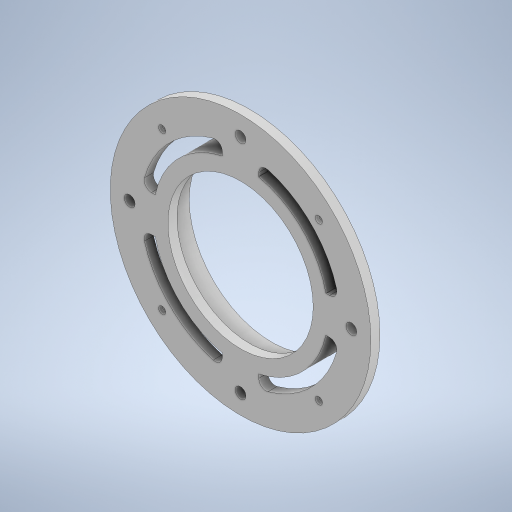
# Autodesk Inventor part: 하단 맨 위부분
Saved by Autodesk Inventor 2023 (Build 270158000, 158)
## iProperties
Created: 2022-06-06
Part Number: 하단 맨 위부분
Material: 일반
Document SubType Name: Modeling
Designer: fly01
Density: 1 g/cm^3
Appearance: 기본값
Author: fly01
Autodesk Inventor part; units mm, degrees
ref_plane "YZ Plane" through (0, 0, 0) normal (1, 0, 0) x (0, 1, 0)
ref_plane "XZ Plane" through (0, 0, 0) normal (0, 1, 0) x (-1, 0, 0)
ref_plane "XY Plane" through (0, 0, 0) normal (0, 0, 1) x (1, 0, 0)
sketch "스케치1" plane through (0, 0, 0) normal (0, 0, 1) x (1, 0, 0)
  circle A0 centre (0, 0) radius 71.7255
  circle A1 centre (0, 0) radius 55
  circle A2 centre (0, 0) radius 61
  circle A3 centre (0, 61) radius 3
  circle A4 centre (-61, 0) radius 3
  circle A5 centre (0, -61) radius 3
  circle A6 centre (61, 0) radius 3
  dimension "d2" = 122
  dimension "d0" = 143.451
  dimension "d1" = 110
  dimension "d3" = 6
  dimension "d6" = 360
  constraints: 6 centre point, 3 coincident, 1 vertical alignment, 11 other
  measures "d0" diameter of A0
  measures "d1" diameter of A1
  measures "d3" diameter of A3
extrude "돌출1" add sketch "스케치1" along normal blind 5 contours A0 | A6 A2 A5 A4 A3
sketch "스케치2" plane through (0, 0, 5) normal (0, 0, 1) x (1, 0, 0)
  circle A0 centre (-43.1335, 43.1335) radius 2
  line L0 (0, 0) -> (-43.1335, 43.1335) construction
  circle A1 centre (0, 61) radius 3 projected
  circle A2 centre (0, 0) radius 61 construction
  line L1 (0, 0) -> (-61, 0) construction
  circle A3 centre (-43.1335, 43.1335) radius 1.25
  circle A4 centre (-43.1335, -43.1335) radius 2
  circle A5 centre (-43.1335, -43.1335) radius 1.25
  circle A6 centre (43.1335, -43.1335) radius 2
  circle A7 centre (43.1335, -43.1335) radius 1.25
  circle A8 centre (43.1335, 43.1335) radius 2
  circle A9 centre (43.1335, 43.1335) radius 1.25
  dimension "d10" = 4
  dimension "d11" = 45
  dimension "d12" = 2.5
  dimension "d15" = 360
  constraints: 9 centre point, 9 coincident, 4 end point, 3 point on circle, 1 horizontal, 21 other
  measures "d10" diameter of A0
  measures "d11" angle of L1 L0
  measures "d12" diameter of A3
extrude "돌출2" cut sketch "스케치2" against normal blind 2 contours A0 | A3 | A4 | A5 | A6 | A7 | A8 | A9
extrude "돌출3" cut sketch "스케치2" against normal blind 5 contours A3 | A5 | A7 | A9
sketch "스케치3" plane through (0, 0, 5) normal (0, 0, 1) x (1, 0, 0)
  circle A0 centre (0, 0) radius 45.25
  circle A1 centre (0, 0) radius 40
  line L0 (-67.4563, 10) -> (-42.5437, 10)
  line L1 (-42.5437, 10) -> (-42.5437, -10)
  line L2 (-42.5437, -10) -> (-67.4563, -10)
  line L3 (-67.4563, -10) -> (-67.4563, 10)
  circle A2 centre (0, 0) radius 55 projected
  line L4 (-67.4563, 10) -> (-42.5437, -10) construction
  line L5 (-42.5437, 10) -> (-67.4563, -10) construction
  point P0 (-55, 0)
  point P1 (-54.0833, 10)
  point P2 (-54.0833, -10)
  point P3 (-44.1312, -10)
  point P4 (-44.1312, 10)
  dimension "d21" = 90.5
  dimension "d22" = 80
  dimension "d23" = 20
  constraints: 12 end point, 2 centre point, 2 coincident, 2 midpoint, 2 parallel, 1 horizontal, 1 perpendicular, 2 other
  measures "d21" diameter of A0
  measures "d22" diameter of A1
  measures "d23" distance between parallel lines of L2 L0
extrude "돌출4" add sketch "스케치3" against normal blind 5 contours A0 L2 L1 L0 | L0 L1 L2 A0
extrude "돌출5" add sketch "스케치3" against normal blind 5 contours A0 L2 A2 L0 picked at (-47.7799, -7.786)
fillet "모깎기1" radius 4 4 edges at (-54.0833, 10, 2.5) (-54.0833, -10, 2.5) (-44.1312, -10, 2.5) (-44.1312, 10, 2.5)
pattern_circular "원형 패턴1" count 4 over 360 about axis through (0, 0, 5) along (0, 0, -1) of "돌출5", "모깎기1"
sketch "스케치4" plane through (0, 0, 0) normal (0, 0, -1) x (-1, 0, 0)
  circle A0 centre (0, 0) radius 48
  circle A1 centre (0, 0) radius 45.25
  dimension "d32" = 96
  dimension "d33" = 90.5
  constraints: 2 centre point, 2 coincident
  measures "d32" diameter of A0
  measures "d33" diameter of A1
extrude "돌출6" add sketch "스케치4" along normal blind 12 and the other way blind 5
